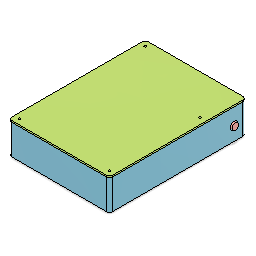
PowerBank (Autodesk Fusion 360 design; units mm, degrees)
Autodesk Fusion 360 part; units mm, degrees
sketch "Sketch1" plane through (0, 0, 0) normal (1, 0, 0) x (0, 0, -1) in component "Batteries"
  circle A0 centre (0, 0) radius 9.25
  circle A1 centre (18.5, 0) radius 9.25
  circle A2 centre (37, 0) radius 9.25
  circle A3 centre (55.5, 0) radius 9.25
  dimension "d3" = 18.5
  dimension "d7" = 55.5
  dimension "d8" = 0
  dimension "d82" = 0
  dimension "d83" = 0
  dimension "d84" = 0
  dimension "d85" = 0
  dimension "d128" = 0
  dimension "d129" = 0
  dimension "d130" = 0
  dimension "d131" = 0
  constraint coincident A0.centre origin
  measures "d3" diameter of A0
extrude "Extrude1" add sketch "Sketch1" along normal blind 65.25 makes body 1 in component "Batteries"
sketch "Sketch1 (2)" plane through (0, 0, 0) normal (0, 1, 0) x (1, 0, 0) in component "Board"
  line L0 (0, 0) -> (57.15, 0)
  line L1 (57.15, 0) -> (57.15, -26.75)
  line L2 (57.15, -26.75) -> (0, -26.75)
  line L3 (0, -26.75) -> (0, 0)
  dimension "d12" = 57.15
  dimension "d13" = 26.75
  dimension "d102" = 0
  dimension "d103" = 0
  dimension "d104" = 0
  dimension "d105" = 0
  dimension "d114" = 0
  dimension "d115" = 0
  dimension "d116" = 0
  dimension "d117" = 0
  dimension "d160" = 0
  dimension "d161" = 0
  dimension "d162" = 0
  dimension "d163" = 0
  dimension "d195" = 0
  dimension "d196" = 0
  dimension "d197" = 0
  dimension "d198" = 0
  dimension "d203" = 0
  dimension "d204" = 0
  dimension "d205" = 0
  dimension "d206" = 0
  constraint horizontal L0
  constraint vertical L1
  constraint horizontal L2
  constraint vertical L3
  constraint coincident L0.start L3.end
  measures "d12" distance of L0.start L0.end
  measures "d13" distance of L0.start L2.end
extrude "Extrude1'" add sketch "Sketch1 (2)" along normal blind 1.05 separate body makes body 2 in component "Board"
sketch "Sketch2" plane through (0, 1.05, 0) normal (0, 1, 0) x (-1, 0, 0) in component "Board"
  line L0 (0, 26.75) -> (-57.15, 26.75)
  line L1 (-57.15, 26.75) -> (-57.15, 0)
  line L2 (-57.15, 0) -> (0, 0)
  line L3 (0, 0) -> (0, 26.75)
  line L4 (-5, 0) -> (-19.6, 0)
  line L5 (-19.6, 0) -> (-19.6, 10)
  line L6 (-19.6, 10) -> (-5, 10)
  line L7 (-5, 10) -> (-5, 0)
  line L8 (0, 0) -> (-5, 0) construction
  line L9 (-19.6, 0) -> (-21.1, 0) construction
  line L10 (-21.1, 0) -> (-28.8, 0)
  line L11 (-28.8, 0) -> (-28.8, 5.8)
  line L12 (-28.8, 5.8) -> (-21.1, 5.8)
  line L13 (-21.1, 5.8) -> (-21.1, 0)
  line L14 (-28.8, 0) -> (-30.3, 0) construction
  line L15 (-30.3, 0) -> (-44.9, 0)
  line L16 (-44.9, 0) -> (-44.9, 10)
  line L17 (-44.9, 10) -> (-30.3, 10)
  line L18 (-30.3, 10) -> (-30.3, 0)
  line L19 (0, 26.75) -> (-4.5, 26.75) construction
  line L20 (-4.5, 26.75) -> (-4.5, 13.75) construction
  line L21 (-4.5, 13.75) -> (0, 13.75) construction
  line L22 (0, 13.75) -> (0, 26.75) construction
  circle A0 centre (-4.5, 13.75) radius 0.75
  line L23 (-57.15, 26.75) -> (-47.15, 26.75) construction
  line L24 (-47.15, 26.75) -> (-47.15, 11.75) construction
  line L25 (-47.15, 11.75) -> (-57.15, 11.75) construction
  line L26 (-57.15, 11.75) -> (-57.15, 26.75) construction
  circle A1 centre (-47.15, 11.75) radius 0.75
  line L27 (-57.15, 0) -> (-56.15, 0) construction
  line L28 (-56.15, 0) -> (-56.15, 3) construction
  line L29 (-56.15, 3) -> (-57.15, 3) construction
  line L30 (-57.15, 3) -> (-57.15, 0) construction
  line L31 (-56.15, 3) -> (-50.25, 3)
  line L32 (-50.25, 3) -> (-50.25, 10.5)
  line L33 (-50.25, 10.5) -> (-56.15, 10.5)
  line L34 (-56.15, 10.5) -> (-56.15, 3)
  dimension "d16" = 14.6
  dimension "d17" = 10
  dimension "d18" = 5
  dimension "d21" = 1.5
  dimension "d22" = 5.8
  dimension "d23" = 7.7
  dimension "d24" = 1.5
  dimension "d25" = 14.6
  dimension "d26" = 10
  dimension "d29" = 4.5
  dimension "d30" = 13
  dimension "d31" = 1.5
  dimension "d32" = 15
  dimension "d33" = 10
  dimension "d34" = 1.5
  dimension "d37" = 1
  dimension "d38" = 3
  dimension "d39" = 5.9
  dimension "d40" = 7.5
  constraint horizontal L4
  constraint vertical L5
  constraint horizontal L6
  constraint vertical L7
  constraint coincident L2 L4.start
  constraint horizontal L8
  constraint coincident L2.end L3.start
  constraint coincident L4.start L7.end
  constraint perpendicular L5 L9
  constraint horizontal L10
  constraint vertical L11
  constraint horizontal L12
  constraint vertical L13
  constraint horizontal L14
  constraint horizontal L15
  constraint vertical L16
  constraint horizontal L17
  constraint vertical L18
  constraint horizontal L19
  constraint vertical L20
  constraint horizontal L21
  constraint vertical L22
  constraint coincident L0.start L3.end
  constraint coincident L20.end L21.start
  constraint horizontal L23
  constraint vertical L24
  constraint horizontal L25
  constraint vertical L26
  constraint coincident L0.end L1.start
  constraint coincident L24.end L25.start
  constraint horizontal L27
  constraint vertical L28
  constraint horizontal L29
  constraint vertical L30
  constraint coincident L1.end L2.start
  constraint horizontal L31
  constraint vertical L32
  constraint horizontal L33
  constraint vertical L34
  measures "d16" distance of L4.start L4.end
  measures "d17" distance of L4.start L6.end
  measures "d18" distance of L2.end L4.start
  measures "d21" distance of L4.end L9.end
  measures "d22" distance of L9.end L12.end
  measures "d23" distance of L9.end L10.end
  measures "d24" distance of L10.end L14.end
  measures "d25" distance of L14.end L15.end
  measures "d26" distance of L14.end L17.end
  measures "d29" distance of L0.start L19.end
  measures "d30" distance of L0.start L21.end
  measures "d31" diameter of A0
  measures "d32" distance of L0.end L25.end
  measures "d33" distance of L0.end L23.end
  measures "d34" diameter of A1
  measures "d37" distance of L1.end L27.end
  measures "d38" distance of L1.end L29.end
  measures "d39" distance of L28.end L31.end
  measures "d40" distance of L28.end L33.end
extrude "Extrude2" add sketch "Sketch2" along normal blind 7.1 separate body contours L2 L4 L5 L6 L7 | L2 L15 L16 L17 L18 | L31 L32 L33 L34 makes body 3 at (9.8667, 1.05, 3.3333) makes body 4 at (35.1667, 1.05, 6.6667) makes body 5 at (56.15, 3.4167, 8) in component "Board"
extrude "Extrude3" add sketch "Sketch2" along normal blind 2.5 separate body contours L2 L10 L11 L12 L13 makes body 6 in component "Board"
extrude "Extrude4" cut sketch "Sketch2" against normal up to surface (1.05 mm away) contours A0 | A1 bodies 2 6 4 3 in component "Board"
sketch "Sketch3" plane through (56.15, 0, 0) normal (1, 0, 0) x (0, 0, -1) in component "Board"
  line L0 (-3, 1.05) -> (-3, 8.15)
  line L1 (-3, 8.15) -> (-10.5, 8.15)
  line L2 (-10.5, 8.15) -> (-10.5, 1.05)
  line L3 (-6.75, 8.15) -> (-6.75, 5.15) construction
  circle A0 centre (-6.75, 5.15) radius 1.75
  line L4 (-10.5, 1.05) -> (-3, 1.05)
  dimension "d41" = 3
  dimension "d42" = 3.5
  constraint vertical L3
  constraint midpoint L1 L3.start
  constraint coincident L3.end A0.centre
  measures "d41" distance of L3.start L3.end
  measures "d42" diameter of A0
extrude "Extrude5" add sketch "Sketch3" along normal blind 1 contours A0 bodies 6 4 2 3 5 in component "Board"
sketch "Sketch4" plane through (0, 0, 0) normal (0, -1, 0) x (1, 0, 0) in component "Board"
  circle A0 centre (4.5, 13.75) radius 0.75
  circle A1 centre (47.15, 11.75) radius 0.75
  line L0 (57.15, 26.75) -> (0, 26.75)
  line L1 (0, 26.75) -> (0, 0)
  line L2 (0, 0) -> (57.15, 0)
  line L3 (57.15, 0) -> (57.15, 26.75)
  line L4 (0, 26.75) -> (9, 26.75) construction
  line L5 (9, 26.75) -> (46, 26.75)
  line L6 (46, 26.75) -> (46, 9.75)
  line L7 (46, 9.75) -> (9, 9.75)
  line L8 (9, 9.75) -> (9, 26.75)
  line L9 (46, 18.25) -> (46, 23.25) construction
  line L10 (46, 18.25) -> (46, 13.25) construction
  line L11 (46, 26.75) -> (38.5, 26.75) construction
  line L12 (46, 9.75) -> (38.5, 9.75) construction
  line L13 (38.5, 9.75) -> (46, 13.25)
  line L14 (46, 23.25) -> (38.5, 26.75)
  dimension "d45" = 9
  dimension "d46" = 37
  dimension "d47" = 17
  dimension "d48" = 5
  dimension "d49" = 5
  dimension "d50" = 7.5
  dimension "d51" = 7.5
  constraint horizontal L4
  constraint coincident L0.end L1.start
  constraint horizontal L5
  constraint vertical L6
  constraint horizontal L7
  constraint vertical L8
  constraint vertical L9
  constraint midpoint L6 L9.start
  constraint vertical L10
  constraint horizontal L11
  constraint horizontal L12
  measures "d45" distance of L0.end L4.end
  measures "d46" distance of L4.end L5.end
  measures "d47" distance of L4.end L7.end
  measures "d48" distance of L9.start L9.end
  measures "d49" distance of L9.start L10.end
  measures "d50" distance of L5.end L11.end
  measures "d51" distance of L6.end L12.end
extrude "Extrude6" add sketch "Sketch4" along normal blind 3.75 contours L0 L5 L6 L7 L8 L13 L14 bodies 2 in component "Board"
sketch "Sketch5" plane through (0, -3.75, 0) normal (0, -1, 0) x (1, 0, 0) in component "Board"
  line L0 (38.5, 9.75) -> (46, 13.25)
  line L1 (46, 13.25) -> (46, 23.25)
  line L2 (46, 23.25) -> (38.5, 26.75)
  line L3 (38.5, 26.75) -> (9, 26.75)
  line L4 (9, 26.75) -> (9, 9.75)
  line L5 (9, 9.75) -> (38.5, 9.75)
  line L6 (38.5, 26.75) -> (38.5, 9.75)
  constraint coincident L2.end L3.start
  constraint coincident L0.start L5.end
extrude "Extrude7" add sketch "Sketch5" along normal blind 1.8 contours L3 L4 L5 L6 bodies 2 in component "Board"
sketch "Sketch1 (3)" plane through (0, 0, 0) normal (0, 1, 0) x (1, 0, 0) in component "BottomCover"
  line L0 (0, 0) -> (74, 0)
  line L1 (74, 0) -> (74, -102)
  line L2 (74, -102) -> (0, -102)
  line L3 (0, -102) -> (0, 0)
  line L4 (0, 0) -> (74, -102) construction
  line L5 (76.5, -104.5) -> (-2.5, -104.5)
  line L6 (-2.5, -104.5) -> (-2.5, 2.5)
  line L7 (-2.5, 2.5) -> (76.5, 2.5)
  line L8 (76.5, 2.5) -> (76.5, -104.5)
  line L9 (76.5, -104.5) -> (-2.5, 2.5) construction
  line L10 (-2.5, -104.5) -> (76.5, 2.5) construction
  point P0 (37, -51)
  dimension "d71" = 74
  dimension "d72" = 102
  dimension "d76" = 79
  dimension "d77" = 107
  dimension "d106" = 0
  dimension "d107" = 0
  dimension "d108" = 0
  dimension "d109" = 0
  dimension "d118" = 0
  dimension "d119" = 0
  dimension "d120" = 0
  dimension "d121" = 0
  dimension "d164" = 0
  dimension "d165" = 0
  dimension "d166" = 0
  dimension "d167" = 0
  dimension "d199" = 0
  dimension "d200" = 0
  dimension "d201" = 0
  dimension "d202" = 0
  dimension "d207" = 0
  dimension "d208" = 0
  dimension "d209" = 0
  dimension "d210" = 0
  constraint horizontal L0
  constraint vertical L1
  constraint horizontal L2
  constraint vertical L3
  constraint coincident L0.start L3.end
  constraint perpendicular L5 L6
  constraint parallel L5 L7
  constraint parallel L6 L8
  constraint horizontal L5
  constraint coincident L9 P0
  constraint coincident L10 P0
  constraint midpoint L4 P0
  measures "d71" distance of L0.start L0.end
  measures "d72" distance of L0.start L2.end
  measures "d76" distance of L6.end L7.end
  measures "d77" distance of L5.end L6.end
extrude "Extrude1''" add sketch "Sketch1 (3)" along normal blind 2.5 separate body contours L0 L1 L2 L3 makes body 7
extrude "Extrude2'" add sketch "Sketch1 (3)" along normal blind 23.5 bodies 7
sketch "Sketch2 (2)" plane through (0, 2.5, 0) normal (0, 1, 0) x (-1, 0, 0) in component "BottomCover"
  line L0 (0, 102) -> (-74, 102)
  line L1 (-74, 102) -> (-74, 0)
  line L2 (-74, 0) -> (0, 0)
  line L3 (0, 0) -> (0, 102)
  line L4 (0, 102) -> (0, 97) construction
  line L5 (0, 97) -> (-74, 97)
  line L6 (0, 97) -> (0, 31.75)
  line L7 (0, 31.75) -> (-74, 31.75)
  dimension "d94" = 5
  dimension "d95" = 65.25
  constraint vertical L4
  constraint coincident L0.start L3.end
  constraint coincident L1 L5.end
  constraint perpendicular L1 L5
  constraint vertical L6
  constraint coincident L1 L7.end
  constraint perpendicular L1 L7
  measures "d94" distance of L0.start L4.end
  measures "d95" distance of L4.end L6.end
extrude "Extrude1'''" add sketch "Sketch2 (2)" along normal blind 6.25 separate body contours L1 L3 L5 L6 L7 makes body 8 in component "BottomCover"
sketch "Sketch3 (2)" plane through (0, 0, 97) normal (0, 0, 1) x (1, 0, 0) in component "BottomCover"
  line L0 (0, 2.5) -> (74, 2.5)
  line L1 (74, 2.5) -> (74, 8.75)
  line L2 (74, 8.75) -> (0, 8.75)
  line L3 (0, 8.75) -> (0, 2.5)
  circle A0 centre (9.25, 11.75) radius 9.25
  circle A1 centre (64.75, 11.75) radius 9.25
  arc A2 (37, 11.75) -> (18.5, 11.75) centre (27.75, 11.75) ccw
  arc A3 (18.5, 11.75) -> (37, 11.75) centre (27.75, 11.75) ccw
  arc A4 (55.5, 11.75) -> (37, 11.75) centre (46.25, 11.75) ccw
  arc A5 (37, 11.75) -> (55.5, 11.75) centre (46.25, 11.75) ccw
extrude "Extrude2''" [suppressed] in component "Batteries"
extrude "Extrude2'''" cut sketch "Sketch3 (2)" against normal blind 65.25 contours L2 A0 | L2 A3 | L2 A5 | L2 A1 picked at (9.8413, 5.8388) picked at (65.8065, 5.6357) bodies 8 in component "BottomCover"
copy_body "CutPasteBodies1" bodies 7 removing the originals makes body 9 in component "BottomCover"
sketch "Sketch5 (2)" plane through (0, 2.5, 0) normal (0, 1, 0) x (-1, 0, 0) in component "BottomCover"
  line L0 (0, 102) -> (-74, 102)
  line L1 (-74, 102) -> (-74, 0)
  line L2 (-74, 0) -> (0, 0)
  line L3 (0, 0) -> (0, 102)
  circle A0 centre (-61, 11.75) radius 0.75
  circle A1 centre (-18.35, 13.75) radius 0.75
  circle A2 centre (-18.35, 13.75) radius 2.25
  circle A3 centre (-61, 11.75) radius 2.25
  dimension "d124" = 1.5
  dimension "d125" = 1.5
  measures "d124" distance of A1
  measures "d125" distance of A0
extrude "Extrude4'" add sketch "Sketch5 (2)" along normal up to surface (3 mm away) contours A2 | A3 bodies 9 in component "BottomCover"
sketch "Sketch6" plane through (0, 2.5, 0) normal (0, 1, 0) x (-1, 0, 0) in component "BottomCover"
  circle A0 centre (-18.35, 13.75) radius 2.25
  line L0 (0, 102) -> (-74, 102)
  line L1 (-74, 102) -> (-74, 0)
  line L2 (-74, 0) -> (0, 0)
  line L3 (0, 0) -> (0, 102)
  circle A1 centre (-61, 11.75) radius 2.25
  circle A2 centre (-74, 102) radius 5
  circle A3 centre (0, 102) radius 5
  circle A4 centre (0, 0) radius 5
  line L4 (-71, 26.75) -> (-13.85, 26.75) construction
  line L5 (-55.5, 31.75) -> (-74, 31.75) construction
  line L6 (-69, 31.0583) -> (-76.5, 31.0583)
  line L7 (-76.5, 31.0583) -> (-76.5, 26.0583)
  line L8 (-76.5, 26.0583) -> (-69, 26.0583)
  line L9 (-69, 26.0583) -> (-69, 31.0583)
  line L10 (-69, 31.0583) -> (-76.5, 26.0583) construction
  line L11 (-76.5, 31.0583) -> (-69, 26.0583) construction
  line L12 (-76.5, 104.5) -> (-76.5, -2.5)
  point P0 (-72.75, 28.5583)
  dimension "d144" = 10
  dimension "d145" = 10
  dimension "d146" = 10
  dimension "d147" = 7.5
  dimension "d148" = 5
  constraint coincident L0.end L1.start
  constraint coincident L0.start L3.end
  constraint coincident L2.end L3.start
  constraint perpendicular L6 L7
  constraint parallel L6 L8
  constraint parallel L7 L9
  constraint horizontal L6
  constraint coincident L10 P0
  constraint coincident L11 P0
  constraint collinear L7 L12
  measures "d144" diameter of A2
  measures "d145" diameter of A3
  measures "d146" diameter of A4
  measures "d147" distance of L7.end L8.end
  measures "d148" distance of L6.end L7.end
extrude "Extrude5'" add sketch "Sketch6" along normal blind 19.55 separate body contours L0 L1 A2 | L0 L3 A3 | L1 L6 L8 L9 | L2 L3 A4 picked at (-70.6836, 101.7628) picked at (-3.2489, 101.2933) picked at (-3.3164, 0.2372) makes body 10 at (4.8591, 15.5333, 100.8212) makes body 11 at (4.9774, 15.5333, 0.4753) makes body 12 at (69.0057, 15.5333, 101.7621) makes body 13 at (70.6667, 9.0167, 31.0583) in component "BottomCover"
fillet "Fillet1" radius 2.5 2 edges at (69, 12.275, 26.0583) (69, 12.275, 31.0583) on bodies 13 in component "BottomCover"
sketch "Sketch7" plane through (0, 0, -2.5) normal (0, 0, -1) x (-1, 0, 0) in component "BottomCover"
  line L0 (-76.5, 0) -> (2.5, 0)
  line L1 (2.5, 0) -> (2.5, 23.5)
  line L2 (2.5, 23.5) -> (-76.5, 23.5)
  line L3 (-76.5, 23.5) -> (-76.5, 0)
  line L4 (-58.75, 6.55) -> (-44.15, 6.55)
  line L5 (-44.15, 6.55) -> (-44.15, 13.65)
  line L6 (-44.15, 13.65) -> (-58.75, 13.65)
  line L7 (-58.75, 13.65) -> (-58.75, 6.55)
  line L8 (-42.65, 6.55) -> (-34.95, 6.55)
  line L9 (-34.95, 6.55) -> (-34.95, 9.05)
  line L10 (-34.95, 9.05) -> (-42.65, 9.05)
  line L11 (-42.65, 9.05) -> (-42.65, 6.55)
  line L12 (-33.45, 6.55) -> (-18.85, 6.55)
  line L13 (-18.85, 6.55) -> (-18.85, 13.65)
  line L14 (-18.85, 13.65) -> (-33.45, 13.65)
  line L15 (-33.45, 13.65) -> (-33.45, 6.55)
  line L16 (-58.75, 13.65) -> (-18.85, 13.65)
  line L17 (-18.85, 13.65) -> (-18.85, 6.55)
  line L18 (-18.85, 6.55) -> (-58.75, 6.55)
  line L19 (-58.75, 6.55) -> (-58.75, 13.65)
  line L20 (-16.85, 4.55) -> (-60.75, 4.55)
  line L21 (-60.75, 4.55) -> (-60.75, 15.65)
  line L22 (-60.75, 15.65) -> (-16.85, 15.65)
  line L23 (-16.85, 15.65) -> (-16.85, 4.55)
  dimension "d154" = -2
  constraint horizontal L16
  constraint vertical L17
  constraint horizontal L18
  constraint vertical L19
  constraint coincident L12.end L13.start
  constraint coincident L6.end L7.start
extrude "Extrude6'" cut sketch "Sketch7" against normal blind 2.5 contours L4 L5 L6 L7 L16 L18 L19 | L8 L9 L10 L11 L18 | L12 L13 L14 L15 L16 L17 L18 bodies 9 10 11 12 13 in component "BottomCover"
sketch "Sketch1 (4)" plane through (76.5, 0, 0) normal (1, 0, 0) x (0, 0, -1)
  line L0 (-104.5, 0) -> (2.5, 0)
  line L1 (2.5, 0) -> (2.5, 23.5)
  line L2 (2.5, 23.5) -> (-104.5, 23.5)
  line L3 (-104.5, 23.5) -> (-104.5, 0)
  circle A0 centre (-6.75, 10.65) radius 1.75 construction
  circle A1 centre (-6.75, 10.65) radius 3.075
  dimension "d157" = 6.15
  constraint concentric A0 A1
  measures "d157" diameter of A1
extrude "Extrude8" cut sketch "Sketch1 (4)" against normal blind 2.5 contours A1 bodies 10 13 12 9 11 in component "BottomCover"
chamfer "Chamfer1" distance 1.25 angle 45 2 edges at (63.0977, 2.5, 12.5636) (20.4477, 2.5, 14.5636) on bodies 9 in component "BottomCover"
sketch "Sketch1 (5)" plane through (0, 23.5, 0) normal (0, 1, 0) x (-1, 0, 0) in component "TopCover"
  line L0 (-74, 102) -> (0, 102)
  line L1 (0, 102) -> (0, 0)
  line L2 (0, 0) -> (-74, 0)
  line L3 (-74, 0) -> (-74, 102)
  line L4 (-76.5, -2.5) -> (2.5, -2.5)
  line L5 (2.5, -2.5) -> (2.5, 104.5)
  line L6 (2.5, 104.5) -> (-76.5, 104.5)
  line L7 (-76.5, 104.5) -> (-76.5, -2.5)
  line L8 (0, 0) -> (-74, 0)
  line L9 (-74, 0) -> (-74, 102)
  line L10 (-74, 102) -> (0, 102)
  line L11 (0, 102) -> (0, 0)
  line L12 (2.5, -2.5) -> (-76.5, -2.5)
  line L13 (-76.5, -2.5) -> (-76.5, 104.5)
  line L14 (-76.5, 104.5) -> (2.5, 104.5)
  line L15 (2.5, 104.5) -> (2.5, -2.5)
  constraint horizontal L8
  constraint vertical L9
  constraint horizontal L10
  constraint vertical L11
  constraint coincident L0.start L3.end
  constraint coincident L1.end L2.start
  constraint horizontal L12
  constraint vertical L13
  constraint horizontal L14
  constraint vertical L15
  constraint coincident L6.end L7.start
  constraint coincident L4.end L5.start
extrude "Extrude1''''" add sketch "Sketch1 (5)" against normal blind 1.25 separate body contours L0 L1 L2 L3 L8 L9 L10 L11 makes body 14 in component "TopCover"
extrude "Extrude2''''" add sketch "Sketch1 (5)" along normal blind 1.25 contours L0 L1 L2 L3 L8 L9 L10 L11 | L4 L5 L6 L7 L12 L13 L14 L15 bodies 14 in component "TopCover"
fillet "Fillet2" radius 2.5 4 edges at (-2.5, 11.75, 104.5) (-2.5, 11.75, -2.5) (76.5, 11.75, -2.5) (76.5, 11.75, 104.5) on bodies 9 in component "BottomCover"
fillet "Fillet1'" radius 2.5 4 edges at (76.5, 24.125, 104.5) (-2.5, 24.125, 104.5) (-2.5, 24.125, -2.5) (76.5, 24.125, -2.5) on bodies 14 in component "TopCover"
sketch "Sketch8" plane through (0, 22.05, 0) normal (0, 1, 0) x (-1, 0, 0) in component "BottomCover"
  arc A0 (-71.5, 26.0583) -> (-71.5, 31.0583) centre (-71.5, 28.5583) ccw
  line L0 (-71.5, 31.0583) -> (-74, 31.0583)
  line L1 (-74, 26.0583) -> (-71.5, 26.0583)
  arc A1 (0, 5) -> (-5, 0) centre (0, 0) ccw construction
  arc A2 (-74, 97) -> (-69, 102) centre (-74, 102) ccw construction
  arc A3 (-5, 102) -> (0, 97) centre (0, 102) ccw construction
  line L2 (0, 0) -> (-3.5355, 3.5355) construction
  line L3 (-69, 28.5583) -> (-74, 28.5644) construction
  line L4 (-74, 102) -> (-70.4645, 98.4645) construction
  line L5 (0, 102) -> (-3.5355, 98.4645) construction
  circle A4 centre (-1.7678, 100.2322) radius 0.75
  circle A5 centre (-1.7678, 1.7678) radius 0.75
  circle A6 centre (-71.5, 28.5583) radius 0.75
  circle A7 centre (-72.2322, 100.2322) radius 0.75
  line L6 (-74, 31.0583) -> (-74, 26.0583)
  line L7 (0, 0) -> (0, 5)
  line L8 (-5, 0) -> (0, 0)
  line L9 (-74, 102) -> (-74, 97)
  line L10 (-69, 102) -> (-74, 102)
  line L11 (0, 102) -> (-5, 102)
  line L12 (0, 97) -> (0, 102)
  dimension "d177" = 1.5
  dimension "d178" = 1.5
  dimension "d179" = 1.5
  dimension "d180" = 1.5
  constraint coincident A1.centre L2.start
  constraint midpoint A1 L2.end
  constraint midpoint A0 L3.start
  constraint coincident A2.centre L4.start
  constraint midpoint A2 L4.end
  constraint coincident A3.centre L5.start
  constraint midpoint A3 L5.end
  constraint midpoint L5 A4.centre
  constraint midpoint L2 A5.centre
  constraint midpoint L4 A7.centre
  constraint coincident A0.centre A6.centre
  measures "d177" diameter of A4
  measures "d178" diameter of A5
  measures "d179" diameter of A6
  measures "d180" diameter of A7
extrude "Extrude10" cut sketch "Sketch8" against normal blind 9.25 contours A4 | A5 | A6 | A7 bodies 11 13 10 12 9 in component "BottomCover"
sketch "Sketch2 (3)" plane through (0, 24.75, 0) normal (0, 1, 0) x (-1, 0, 0) in component "TopCover"
  arc A0 (-76.5, 0) -> (-74, -2.5) centre (-74, 0) ccw
  line L0 (-74, -2.5) -> (0, -2.5)
  arc A1 (0, -2.5) -> (2.5, 0) centre (0, 0) ccw
  line L1 (2.5, 0) -> (2.5, 102)
  arc A2 (2.5, 102) -> (0, 104.5) centre (0, 102) ccw
  line L2 (0, 104.5) -> (-74, 104.5)
  arc A3 (-74, 104.5) -> (-76.5, 102) centre (-74, 102) ccw
  line L3 (-76.5, 102) -> (-76.5, 0)
  circle A4 centre (-1.7678, 1.7678) radius 0.75
  circle A5 centre (-1.7678, 100.2322) radius 0.75
  circle A6 centre (-72.2322, 100.2322) radius 0.75
  circle A7 centre (-71.5, 28.5583) radius 0.75
extrude "Extrude3'" cut sketch "Sketch2 (3)" against normal up to surface (2.5 mm away) contours A4 | A5 | A6 | A7 bodies 14 in component "TopCover"
sketch "Sketch10" plane through (0, 0, 0) normal (0, -1, 0) x (1, 0, 0) in component "BottomCover"
  arc A0 (76.5, 102) -> (74, 104.5) centre (74, 102) ccw
  line L0 (74, 104.5) -> (0, 104.5)
  arc A1 (0, 104.5) -> (-2.5, 102) centre (0, 102) ccw
  line L1 (-2.5, 102) -> (-2.5, 0)
  arc A2 (-2.5, 0) -> (0, -2.5) centre (0, 0) ccw
  line L2 (0, -2.5) -> (74, -2.5)
  arc A3 (74, -2.5) -> (76.5, 0) centre (74, 0) ccw
  line L3 (76.5, 0) -> (76.5, 102)
  line L4 (22.85, 26.75) -> (22.85, 9.75)
  line L5 (22.85, 9.75) -> (52.35, 9.75)
  line L6 (52.35, 9.75) -> (52.35, 26.75)
  line L7 (52.35, 26.75) -> (22.85, 26.75)
extrude "Extrude12" cut sketch "Sketch10" against normal blind 2.5 contours L4 L5 L6 L7 bodies 11 13 9 10 12 in component "BottomCover"
sketch "Sketch12" plane through (0, 0, 0) normal (0, 0, 1) x (1, 0, 0) in component "BottomCover"
  line L0 (58.75, 6.55) -> (44.15, 6.55)
  line L1 (44.15, 6.55) -> (44.15, 13.65)
  line L2 (44.15, 13.65) -> (58.75, 13.65)
  line L3 (58.75, 13.65) -> (58.75, 6.55)
  line L4 (42.65, 6.55) -> (34.95, 6.55)
  line L5 (34.95, 6.55) -> (34.95, 9.05)
  line L6 (34.95, 9.05) -> (42.65, 9.05)
  line L7 (42.65, 9.05) -> (42.65, 6.55)
  line L8 (33.45, 6.55) -> (18.85, 6.55)
  line L9 (18.85, 6.55) -> (18.85, 13.65)
  line L10 (18.85, 13.65) -> (33.45, 13.65)
  line L11 (33.45, 13.65) -> (33.45, 6.55)
  line L12 (0, 2.5) -> (74, 2.5)
  line L13 (74, 2.5) -> (74, 23.5)
  line L14 (74, 23.5) -> (0, 23.5)
  line L15 (0, 23.5) -> (0, 2.5)
  line L16 (22.85, 2.5) -> (52.35, 2.5)
  line L17 (52.35, 2.5) -> (22.85, 2.5)
  line L18 (64.5, 2.5) -> (57.5, 2.5)
  line L19 (74, 2.5) -> (0, 2.5)
  line L20 (0, 2.5) -> (74, 2.5)
  line L21 (21.85, 2.5) -> (14.85, 2.5)
  line L22 (16.85, 15.65) -> (16.85, 4.55)
  line L23 (60.75, 15.65) -> (16.85, 15.65)
  line L24 (16.85, 4.55) -> (60.75, 4.55)
  line L25 (60.75, 4.55) -> (60.75, 15.65)
extrude "Extrude13" cut sketch "Sketch12" against normal blind 1 contours L22 L23 L24 L25 bodies 13 12 10 9 11 in component "BottomCover"
move_face "OffsetFaces1" offset 1 3 faces at (9.8667, 5.7833, 0) (26.2333, 1.8833, 0) (40.0333, 3.4167, 0) on bodies 3 4 6 in component "Board"
sketch "Sketch1 (6)" plane through (74, 0, 0) normal (-1, 0, 0) x (0, 0, 1) in component "Knob"
  circle A0 centre (6.75, 10.65) radius 3.075
  line L0 (0, 2.5) -> (102, 2.5)
  line L1 (102, 2.5) -> (102, 23.5)
  line L2 (102, 23.5) -> (0, 23.5)
  line L3 (0, 23.5) -> (0, 2.5)
  circle A1 centre (6.75, 10.65) radius 3.075 construction
  circle A2 centre (6.75, 10.65) radius 4.075
  circle A3 centre (6.75, 10.65) radius 2.575
  dimension "d211" = 1
  dimension "d214" = -0.5
extrude "Extrude1'''''" add sketch "Sketch1 (6)" along normal up to surface (2.5 mm away) separate body contours A0 | A2 | A3 makes body 15 in component "Knob"
extrude "Extrude2'''''" add sketch "Sketch1 (6)" against normal blind 3.5 contours A3 bodies 15 in component "Knob"
extrude "Extrude14" cut sketch "Sketch7" against normal blind 0.5 contours L5 L9 L10 L11 L15 L16 L18 | L20 L21 L22 L23 bodies 12 10 9 11 13 in component "BottomCover"
move_face "OffsetFaces1'" offset -8.25 1 faces at (70.6663, 2.5, 28.5581) on bodies 13 in component "BottomCover"
move_face "OffsetFaces1''" offset -0.1 4 faces at (74, 23.0833, 34) (24.6667, 22.6667, 0) (49.3333, 22.6667, 102) (0, 23.0833, 68) on bodies 14 in component "TopCover"
sketch "Sketch1 (7)" plane through (0, -0.05, 0) normal (0, -1, 0) x (1, 0, 0) in component "DisplayCover"
  line L0 (22.85, 26.75) -> (22.85, 9.75)
  line L1 (22.85, 9.75) -> (52.35, 9.75)
  line L2 (52.35, 9.75) -> (52.35, 26.75)
  line L3 (52.35, 26.75) -> (22.85, 26.75)
  line L4 (22.85, 26.75) -> (52.35, 9.75) construction
  line L5 (50.6, 24.25) -> (24.6, 24.25)
  line L6 (24.6, 24.25) -> (24.6, 12.25)
  line L7 (24.6, 12.25) -> (50.6, 12.25)
  line L8 (50.6, 12.25) -> (50.6, 24.25)
  line L9 (50.6, 24.25) -> (24.6, 12.25) construction
  line L10 (24.6, 24.25) -> (50.6, 12.25) construction
  line L11 (57.6, 31.25) -> (17.6, 31.25)
  line L12 (17.6, 31.25) -> (17.6, 5.25)
  line L13 (17.6, 5.25) -> (57.6, 5.25)
  line L14 (57.6, 5.25) -> (57.6, 31.25)
  point P0 (37.6, 18.25)
  dimension "d229" = 26
  dimension "d230" = 12
  dimension "d231" = 7
  constraint coincident L0.start L3.end
  constraint coincident L1.end L2.start
  constraint perpendicular L5 L6
  constraint parallel L5 L7
  constraint parallel L6 L8
  constraint horizontal L5
  constraint coincident L9 P0
  constraint coincident L10 P0
  constraint midpoint L4 P0
  measures "d229" distance of L6.end L7.end
  measures "d230" distance of L5.end L6.end
extrude "Extrude1''''''" add sketch "Sketch1 (7)" along normal blind 1.25 separate body contours L0 L1 L2 L3 | L11 L12 L13 L14 makes body 16 in component "DisplayCover"
chamfer "Chamfer1'" distance 1 angle 45 2 edges at (50.6, -1.3, 18.25) (24.6, -1.3, 18.25) on bodies 16 in component "DisplayCover"
chamfer "Chamfer2" distance 1 angle 45 2 edges at (37.6, -1.3, 24.25) (37.6, -1.3, 12.25) on bodies 16 in component "DisplayCover"
chamfer "Chamfer3" distance 1.2 angle 45 4 edges at (57.6, -1.3, 18.25) (37.6, -1.3, 5.25) (17.6, -1.3, 18.25) (37.6, -1.3, 31.25) on bodies 16 in component "DisplayCover"
fillet "Fillet1''" radius 2.5 4 edges at (37.6, -1.3, 30.05) (18.8, -1.3, 18.25) (56.4, -1.3, 18.25) (37.6, -1.3, 6.45) on bodies 16 in component "DisplayCover"
component "Batteries" placed x (0, 0, 1) y (0, 1, 0) z (-1, 0, 0) at (9.25, 11.75, 31.75)
component "Board" placed x (1, 0, 0) y (0, 1, 0) z (0, 0, 1) at (13.85, 5.5, 0)
component "BottomCover" placed x (1, 0, 0) y (0, 1, 0) z (0, 0, 1) at (0, 0, 0)
component "TopCover" placed x (1, 0, 0) y (0, 1, 0) z (0, 0, 1) at (0, 0, 0)
component "Knob" placed x (1, 0, 0) y (0, 1, 0) z (0, 0, 1) at (0, 0, 0)
component "DisplayCover" placed x (1, 0, 0) y (0, 1, 0) z (0, 0, 1) at (0, 0, 0)
equation "batteryDiam = 18.5 mm"
equation "batteryLength = 65.25 mm"
equation "d3 = batteryDiam"
equation "d5 = batteriesCount"
equation "d7 = batteryDiam * ( batteriesCount - 1 )"
equation "batteriesCount = 4"
equation "d10 = batteryLength"
equation "d12 = boardLength"
equation "d13 = boardWidth"
equation "d71 = batteryDiam * 4"
equation "d72 = batteryLength + 10 mm + boardWidth"
equation "wallThickness = 2.5 mm"
equation "boardWidth = 26.75 mm"
equation "boardLength = 57.15 mm"
equation "d76 = batteryDiam * batteriesCount + wallThickness * 2"
equation "d77 = batteryLength + 10 mm + boardWidth + wallThickness * 2"
equation "d78 = wallThickness"
equation "d80 = wallThickness + batteryDiam + wallThickness"
equation "d92 = -batteryDiam / 2 - wallThickness"
equation "d95 = batteryLength"
equation "d96 = batteryDiam / 2 - 3 mm"
equation "d98 = -batteryLength"
equation "d100 = -batteryLength"
equation "d147 = wallThickness * 3"
equation "d149 = batteryDiam + wallThickness / 2 - 0.2 mm"
equation "d151 = wallThickness"
equation "d152 = -wallThickness"
equation "d158 = -wallThickness"
equation "d168 = wallThickness / 2"
equation "d173 = wallThickness / 2"
equation "d175 = wallThickness"
equation "d176 = wallThickness"
equation "d181 = -batteryDiam / 2"
equation "d189 = -wallThickness"
equation "d193 = -wallThickness / 2"
equation "d215 = -wallThickness - 1 mm"
equation "d219 = -batteryDiam / 2 + 1 mm"
equation "d232 = wallThickness / 2"
equation "d237 = wallThickness"
